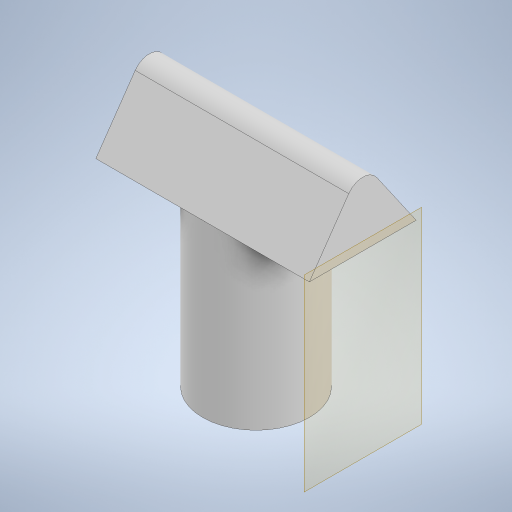
# Autodesk Inventor part: rotator_flat
Saved by Autodesk Inventor 2023.1 (Build 271208000, 208)
## iProperties
Created: 2022-10-07
Part Number: rotator_flat
Material: Generic
Document SubType Name: Modeling
Designer: swang
Density: 1 g/cm^3
Appearance: Default
Author: swang
## iProperties of the stored document rotator_round_3DPrint.ipt
Created: 2022-10-07
Part Number: rotator_round_3DPrint
Material: Generic
Document SubType Name: Modeling
Designer: swang
Density: 1 g/cm^3
Appearance: Default
Author: swang
Autodesk Inventor part; units mm, degrees
ref_plane "XZ Plane" through (0, 0, 0) normal (0, 1, 0) x (-1, 0, 0)
ref_plane "XY Plane" through (0, 0, 0) normal (0, 0, 1) x (1, 0, 0)
sketch "Sketch1" plane through (0, 0, 0) normal (0, 1, 0) x (-1, 0, 0)
  circle A0 centre (0, 0) radius 25
  dimension "d0" = 50
  constraints: 1 centre point, 1 coincident
  measures "d0" diameter of A0
extrude "Extrusion1" add sketch "Sketch1" along normal blind 80
ref_plane "Work Plane3" through (50, 0, 0) normal (1, 0, 0) x (0, 1, 0)
sketch "Sketch7" plane through (50, 0, 0) normal (1, 0, 0) x (0, 1, 0)
  line L0 (80, -25) -> (80, 25) projected
  line L1 (80, 25) -> (80, -25)
  line L2 (80, -25) -> (106.5602, -6.573)
  line L3 (106.5602, 6.573) -> (80, 25)
  arc A0 (106.5602, -6.573) -> (106.5602, 6.573) centre (102, 0) ccw
  point P0 (0, 0)
  point P1 (110, 0)
  dimension "d23" = 8
  dimension "d24" = 30
  constraints: 6 end point, 3 point on circle, 2 tangent, 1 centre point, 1 collinear
  measures "d23" radius of A0
  measures "d24" distance from line of L0 point (110, 0)
extrude "Extrusion5" add sketch "Sketch7" against normal blind 100
body "Solid1"
